Autodesk Fusion 360 part; units mm, degrees
(part 4 of 5)
sketch "Skizze60" plane through (0, 0, 0) normal (0, -1, 0) x (1, 0, 0)
  arc A0 (-6.1259, 60.1453) -> (-6.4721, 59.7023) centre (0, 55) ccw
  arc A1 (-6.4721, 59.7023) -> (-6.8553, 59.1236) centre (-6.6397, 59.397) ccw
  arc A2 (-6.8553, 59.1236) -> (-7.1281, 58.6319) centre (0, 55) ccw
  arc A3 (-7.1281, 58.6319) -> (-7.416, 58.0005) centre (-7.2458, 58.3042) ccw
  arc A4 (-7.416, 58.0005) -> (-7.6085, 57.4721) centre (0, 55) ccw
  arc A5 (-7.6085, 57.4721) -> (-7.7941, 56.8034) centre (-7.6734, 57.13) ccw
  arc A6 (-7.7941, 56.8034) -> (-7.9015, 56.2515) centre (0, 55) ccw
  arc A7 (-7.9015, 56.2515) -> (-7.9802, 55.5619) centre (-7.9122, 55.9034) ccw
  arc A8 (-7.9802, 55.5619) -> (-8, 55) centre (0, 55) ccw
  arc A9 (-8, 55) -> (-7.9699, 54.3066) centre (-7.9561, 54.6546) ccw
  arc A10 (-7.9699, 54.3066) -> (-7.9015, 53.7485) centre (0, 55) ccw
  arc A11 (-7.9015, 53.7485) -> (-7.7633, 53.0684) centre (-7.8041, 53.4142) ccw
  arc A12 (-7.7633, 53.0684) -> (-7.6085, 52.5279) centre (0, 55) ccw
  arc A13 (-7.6085, 52.5279) -> (-7.3656, 51.8777) centre (-7.46, 52.2129) ccw
  arc A14 (-7.3656, 51.8777) -> (-7.1281, 51.3681) centre (0, 55) ccw
  arc A15 (-7.1281, 51.3681) -> (-6.7864, 50.764) centre (-6.9321, 51.0802) ccw
  arc A16 (-6.7864, 50.764) -> (-6.4721, 50.2977) centre (0, 55) ccw
  arc A17 (-6.4721, 50.2977) -> (-6.0402, 49.7545) centre (-6.2336, 50.0441) ccw
  arc A18 (-6.0402, 49.7545) -> (-5.6569, 49.3431) centre (0, 55) ccw
  arc A19 (-5.6569, 49.3431) -> (-5.1453, 48.8741) centre (-5.3816, 49.1299) ccw
  arc A20 (-5.1453, 48.8741) -> (-4.7023, 48.5279) centre (0, 55) ccw
  arc A21 (-4.7023, 48.5279) -> (-4.1236, 48.1447) centre (-4.397, 48.3603) ccw
  arc A22 (-4.1236, 48.1447) -> (-3.6319, 47.8719) centre (0, 55) ccw
  arc A23 (-3.6319, 47.8719) -> (-3.0005, 47.584) centre (-3.3042, 47.7542) ccw
  arc A24 (-3.0005, 47.584) -> (-2.4721, 47.3915) centre (0, 55) ccw
  arc A25 (-2.4721, 47.3915) -> (-1.8034, 47.2059) centre (-2.13, 47.3266) ccw
  arc A26 (-1.8034, 47.2059) -> (-1.2515, 47.0985) centre (0, 55) ccw
  arc A27 (-1.2515, 47.0985) -> (-0.5619, 47.0198) centre (-0.9034, 47.0878) ccw
  arc A28 (-0.5619, 47.0198) -> (0, 47) centre (0, 55) ccw
  arc A29 (0, 47) -> (0.6934, 47.0301) centre (0.3454, 47.0439) ccw
  arc A30 (0.6934, 47.0301) -> (1.2515, 47.0985) centre (0, 55) ccw
  arc A31 (1.2515, 47.0985) -> (1.9316, 47.2367) centre (1.5858, 47.1959) ccw
  arc A32 (1.9316, 47.2367) -> (2.4721, 47.3915) centre (0, 55) ccw
  arc A33 (2.4721, 47.3915) -> (3.1223, 47.6344) centre (2.7871, 47.54) ccw
  arc A34 (3.1223, 47.6344) -> (3.6319, 47.8719) centre (0, 55) ccw
  arc A35 (3.6319, 47.8719) -> (4.236, 48.2136) centre (3.9198, 48.0679) ccw
  arc A36 (4.236, 48.2136) -> (4.7023, 48.5279) centre (0, 55) ccw
  arc A37 (4.7023, 48.5279) -> (5.2455, 48.9598) centre (4.9559, 48.7664) ccw
  arc A38 (5.2455, 48.9598) -> (5.6569, 49.3431) centre (0, 55) ccw
  arc A39 (5.6569, 49.3431) -> (6.1259, 49.8547) centre (5.8701, 49.6184) ccw
  arc A40 (6.1259, 49.8547) -> (6.4721, 50.2977) centre (0, 55) ccw
  arc A41 (6.4721, 50.2977) -> (6.8553, 50.8764) centre (6.6397, 50.603) ccw
  arc A42 (6.8553, 50.8764) -> (7.1281, 51.3681) centre (0, 55) ccw
  arc A43 (7.1281, 51.3681) -> (7.416, 51.9995) centre (7.2458, 51.6958) ccw
  arc A44 (7.416, 51.9995) -> (7.6085, 52.5279) centre (0, 55) ccw
  arc A45 (7.6085, 52.5279) -> (7.7941, 53.1966) centre (7.6734, 52.87) ccw
  arc A46 (7.7941, 53.1966) -> (7.9015, 53.7485) centre (0, 55) ccw
  arc A47 (7.9015, 53.7485) -> (7.9802, 54.4381) centre (7.9122, 54.0966) ccw
  arc A48 (7.9802, 54.4381) -> (8, 55) centre (0, 55) ccw
  arc A49 (8, 55) -> (7.9699, 55.6934) centre (7.9561, 55.3454) ccw
  arc A50 (7.9699, 55.6934) -> (7.9015, 56.2515) centre (0, 55) ccw
  arc A51 (7.9015, 56.2515) -> (7.7633, 56.9316) centre (7.8041, 56.5858) ccw
  arc A52 (7.7633, 56.9316) -> (7.6085, 57.4721) centre (0, 55) ccw
  arc A53 (7.6085, 57.4721) -> (7.3656, 58.1223) centre (7.46, 57.7871) ccw
  arc A54 (7.3656, 58.1223) -> (7.1281, 58.6319) centre (0, 55) ccw
  arc A55 (7.1281, 58.6319) -> (6.7864, 59.236) centre (6.9321, 58.9198) ccw
  arc A56 (6.7864, 59.236) -> (6.4721, 59.7023) centre (0, 55) ccw
  arc A57 (6.4721, 59.7023) -> (6.0402, 60.2455) centre (6.2336, 59.9559) ccw
  arc A58 (6.0402, 60.2455) -> (5.6569, 60.6569) centre (0, 55) ccw
  arc A59 (5.6569, 60.6569) -> (5.1453, 61.1259) centre (5.3816, 60.8701) ccw
  arc A60 (5.1453, 61.1259) -> (4.7023, 61.4721) centre (0, 55) ccw
  arc A61 (4.7023, 61.4721) -> (4.1236, 61.8553) centre (4.397, 61.6397) ccw
  arc A62 (4.1236, 61.8553) -> (3.6319, 62.1281) centre (0, 55) ccw
  arc A63 (3.6319, 62.1281) -> (3.0005, 62.416) centre (3.3042, 62.2458) ccw
  arc A64 (3.0005, 62.416) -> (2.4721, 62.6085) centre (0, 55) ccw
  arc A65 (2.4721, 62.6085) -> (1.8034, 62.7941) centre (2.13, 62.6734) ccw
  arc A66 (1.8034, 62.7941) -> (1.2515, 62.9015) centre (0, 55) ccw
  arc A67 (1.2515, 62.9015) -> (0.5619, 62.9802) centre (0.9034, 62.9122) ccw
  arc A68 (0.5619, 62.9802) -> (0, 63) centre (0, 55) ccw
  arc A69 (0, 63) -> (-0.6934, 62.9699) centre (-0.3454, 62.9561) ccw
  arc A70 (-0.6934, 62.9699) -> (-1.2515, 62.9015) centre (0, 55) ccw
  arc A71 (-1.2515, 62.9015) -> (-1.9316, 62.7633) centre (-1.5858, 62.8041) ccw
  arc A72 (-1.9316, 62.7633) -> (-2.4721, 62.6085) centre (0, 55) ccw
  arc A73 (-2.4721, 62.6085) -> (-3.1223, 62.3656) centre (-2.7871, 62.46) ccw
  arc A74 (-3.1223, 62.3656) -> (-3.6319, 62.1281) centre (0, 55) ccw
  arc A75 (-3.6319, 62.1281) -> (-4.236, 61.7864) centre (-3.9198, 61.9321) ccw
  arc A76 (-4.236, 61.7864) -> (-4.7023, 61.4721) centre (0, 55) ccw
  arc A77 (-4.7023, 61.4721) -> (-5.2455, 61.0402) centre (-4.9559, 61.2336) ccw
  arc A78 (-5.2455, 61.0402) -> (-5.6569, 60.6569) centre (0, 55) ccw
  arc A79 (-5.6569, 60.6569) -> (-6.1259, 60.1453) centre (-5.8701, 60.3816) ccw
  circle A80 centre (0, 55) radius 8
  constraint concentric A0 A80
extrude "Extrusion65" add sketch "Skizze60" along normal blind 1 contours A0 A2 A4 A6 A8 A10 A12 A14 A16 A18 A20 A22 A24 A26 A28 A30 A32 A34 A36 A38 A40 A42 A44 A46 A48 A50 A52 A54 A56 A58 A60 A62 A64 A66 A68 A70 A72 A74 A76 A78 A80 bodies 3
chamfer "Fase2" distance 1 angle 45 1 edges at (-7.4586, -1, 52.1071) on bodies 3
sketch "Skizze61" plane through (0, 0, 27.5) normal (0, 0, 1) x (1, 0, 0)
  line L0 (-32.5, 0) -> (32.5, 0)
  line L1 (32.5, 0) -> (32.5, 16)
  line L2 (32.5, 16) -> (-32.5, 16)
  line L3 (-32.5, 16) -> (-32.5, 0)
  line L4 (-9.4118, 6.9027) -> (-15.8397, 14.5631)
  arc A0 (-15.8397, 14.5631) -> (-18.1378, 12.6348) centre (-16.9888, 13.599) ccw
  line L5 (-18.1378, 12.6348) -> (-11.71, 4.9743)
  arc A1 (-11.71, 4.9743) -> (-9.4118, 6.9027) centre (-10.5609, 5.9385) ccw
  line L6 (-10.5609, 5.9385) -> (-16.9888, 13.599) construction
  line L7 (-9.1378, 12.6348) -> (-2.71, 4.9743)
  arc A2 (-6.8397, 14.5631) -> (-9.1378, 12.6348) centre (-7.9888, 13.599) ccw
  line L8 (-0.4118, 6.9027) -> (-6.8397, 14.5631)
  arc A3 (-2.71, 4.9743) -> (-0.4118, 6.9027) centre (-1.5609, 5.9385) ccw
  line L9 (-0.1378, 12.6348) -> (6.29, 4.9743)
  arc A4 (2.1603, 14.5631) -> (-0.1378, 12.6348) centre (1.0112, 13.599) ccw
  line L10 (8.5882, 6.9027) -> (2.1603, 14.5631)
  arc A5 (6.29, 4.9743) -> (8.5882, 6.9027) centre (7.4391, 5.9385) ccw
  line L11 (8.8622, 12.6348) -> (15.29, 4.9743)
  arc A6 (11.1603, 14.5631) -> (8.8622, 12.6348) centre (10.0112, 13.599) ccw
  line L12 (17.5882, 6.9027) -> (11.1603, 14.5631)
  arc A7 (15.29, 4.9743) -> (17.5882, 6.9027) centre (16.4391, 5.9385) ccw
  dimension "d317" = 3
  dimension "d320" = 27
  dimension "d321" = 0
  constraint tangent L4 A0
  constraint tangent A0 L5
  constraint parallel L4 L5
  constraint tangent L5 A1
  constraint tangent L4 A1
  measures "d317" diameter of A0
extrude "Extrusion66" cut sketch "Skizze61" against normal blind 2 contours L4 A0 L5 A1 | L7 A2 L8 A3 | L9 A4 L10 A5 | L11 A6 L12 A7 bodies 1
extrude "Extrusion67" cut 1 faces at (0.4189, 1, 54.1158) along direction (0, -1, 0) blind 1 on bodies 3 bodies 3
sketch "Skizze62" plane through (0, 10.5, 0) normal (0, 1, 0) x (-1, 0, 0)
  arc A0 (-3.1, 55) -> (1.4484, 57.7408) centre (0, 55) ccw
  line L0 (-3.1, 55) -> (1.4484, 57.7408)
  circle A1 centre (0, 55) radius 4.5
  circle A2 centre (0, 55) radius 3.1
  constraint concentric A0 A2
extrude "Extrusion68" add sketch "Skizze62" along normal blind 3 bodies 3
sketch "Skizze63" plane through (0, 47, 0) normal (0, 1, 0) x (-1, 0, 0)
  line L0 (-20.5, -7.58) -> (-20.5, -6.3514)
  arc A0 (-20.5, -4.3514) -> (-20.5, -6.3514) centre (-20.5, -5.3514) ccw
  line L1 (-20.5, -4.3514) -> (-12.5, -4.3514)
  arc A1 (-12.5, -6.3514) -> (-12.5, -4.3514) centre (-12.5, -5.3514) ccw
  line L2 (-12.5, -6.3514) -> (-12.5, -7.58)
  line L3 (-12.5, -7.58) -> (-20.5, -7.58)
  circle A2 centre (3.5, 16) radius 6.5
  line L4 (21.5, -1.5) -> (21.5, -23.5)
  line L5 (21.5, -23.5) -> (-5.5, -23.5)
  line L6 (-5.5, -23.5) -> (-5.5, -1.5)
  line L7 (-5.5, -1.5) -> (21.5, -1.5)
  line L8 (-37.3325, 4.5) -> (-48.5, 4.5)
  arc A3 (-48.5, 7.5) -> (-48.5, 4.5) centre (-48.5, 6) ccw
  line L9 (-48.5, 7.5) -> (-37.3325, 7.5)
  arc A4 (-37.3325, 4.5) -> (-37.3325, 7.5) centre (-37.3325, 6) ccw
  line L10 (-12.5, 2.5057) -> (-20.5, 2.5057)
  arc A5 (-20.5, 4.5057) -> (-20.5, 2.5057) centre (-20.5, 3.5057) ccw
  line L11 (-20.5, 4.5057) -> (-12.5, 4.5057)
  arc A6 (-12.5, 2.5057) -> (-12.5, 4.5057) centre (-12.5, 3.5057) ccw
  line L12 (-12.5, -15.2086) -> (-20.5, -15.2086)
  arc A7 (-20.5, -13.2086) -> (-20.5, -15.2086) centre (-20.5, -14.2086) ccw
  line L13 (-20.5, -13.2086) -> (-12.5, -13.2086)
  arc A8 (-12.5, -15.2086) -> (-12.5, -13.2086) centre (-12.5, -14.2086) ccw
  arc A9 (34, 7.5) -> (34, 4.5) centre (34, 6) ccw
  line L14 (34, 7.5) -> (45, 7.5)
  arc A10 (45, 4.5) -> (45, 7.5) centre (45, 6) ccw
  line L15 (45, 4.5) -> (34, 4.5)
  arc A11 (34, -10.5) -> (34, -13.5) centre (34, -12) ccw
  line L16 (34, -10.5) -> (45, -10.5)
  arc A12 (45, -13.5) -> (45, -10.5) centre (45, -12) ccw
  line L17 (45, -13.5) -> (34, -13.5)
  arc A13 (34, 13.5) -> (34, 10.5) centre (34, 12) ccw
  line L18 (34, 13.5) -> (45, 13.5)
  arc A14 (45, 10.5) -> (45, 13.5) centre (45, 12) ccw
  line L19 (45, 10.5) -> (34, 10.5)
  line L20 (-12.5, -10.78) -> (-20.5, -10.78)
  arc A15 (-20.5, -8.78) -> (-20.5, -10.78) centre (-20.5, -9.78) ccw
  line L21 (-20.5, -8.78) -> (-12.5, -8.78)
  arc A16 (-12.5, -10.78) -> (-12.5, -8.78) centre (-12.5, -9.78) ccw
  line L22 (-20.5, 8.9343) -> (-12.5, 8.9343)
  arc A17 (-12.5, 6.9343) -> (-12.5, 8.9343) centre (-12.5, 7.9343) ccw
  line L23 (-12.5, 6.9343) -> (-20.5, 6.9343)
  arc A18 (-20.5, 8.9343) -> (-20.5, 6.9343) centre (-20.5, 7.9343) ccw
  line L24 (-37.3325, -1.5) -> (-48.5, -1.5)
  arc A19 (-48.5, 1.5) -> (-48.5, -1.5) centre (-48.5, 0) ccw
  line L25 (-48.5, 1.5) -> (-37.3325, 1.5)
  arc A20 (-37.3325, -1.5) -> (-37.3325, 1.5) centre (-37.3325, 0) ccw
  arc A21 (-20.8852, 0) -> (-20.5, -1.9228) centre (-20.5, -0.9228) ccw
  line L26 (-20.8852, 0) -> (-12.1148, 0)
  arc A22 (-12.5, -1.9228) -> (-12.1148, 0) centre (-12.5, -0.9228) ccw
  line L27 (-12.5, -1.9228) -> (-20.5, -1.9228)
  line L28 (-12.5, -19.6371) -> (-20.5, -19.6371)
  arc A23 (-20.5, -17.6371) -> (-20.5, -19.6371) centre (-20.5, -18.6371) ccw
  line L29 (-20.5, -17.6371) -> (-12.5, -17.6371)
  arc A24 (-12.5, -19.6371) -> (-12.5, -17.6371) centre (-12.5, -18.6371) ccw
  line L30 (34, 1.5) -> (45, 1.5)
  arc A25 (45, -1.5) -> (45, 1.5) centre (45, 0) ccw
  line L31 (45, -1.5) -> (34, -1.5)
  arc A26 (34, 1.5) -> (34, -1.5) centre (34, 0) ccw
  arc A27 (34, -4.5) -> (34, -7.5) centre (34, -6) ccw
  line L32 (34, -4.5) -> (45, -4.5)
  arc A28 (45, -7.5) -> (45, -4.5) centre (45, -6) ccw
  line L33 (45, -7.5) -> (34, -7.5)
  line L34 (-12.5, -24.0657) -> (-20.5, -24.0657)
  arc A29 (-20.5, -22.0657) -> (-20.5, -24.0657) centre (-20.5, -23.0657) ccw
  line L35 (-20.5, -22.0657) -> (-12.5, -22.0657)
  arc A30 (-12.5, -24.0657) -> (-12.5, -22.0657) centre (-12.5, -23.0657) ccw
  line L36 (-37.3325, -7.5) -> (-48.5, -7.5)
  arc A31 (-48.5, -4.5) -> (-48.5, -7.5) centre (-48.5, -6) ccw
  line L37 (-48.5, -4.5) -> (-37.3325, -4.5)
  arc A32 (-37.3325, -7.5) -> (-37.3325, -4.5) centre (-37.3325, -6) ccw
  line L38 (22.3, -10.5) -> (30, -10.5)
  line L39 (30, -10.5) -> (30, -18.5)
  line L40 (30, -18.5) -> (22.3, -18.5)
  line L41 (22.3, -18.5) -> (22.3, -10.5)
  line L42 (-32.5, 27.5) -> (-32.5, 14.5)
  arc A33 (-36, 11) -> (-32.5, 14.5) centre (-36, 14.5) ccw
  line L43 (-36, 11) -> (-56.5, 11)
  line L44 (-56.5, 11) -> (-56.5, -11)
  line L45 (-56.5, -11) -> (-36, -11)
  arc A34 (-32.5, -14.5) -> (-36, -11) centre (-36, -14.5) ccw
  line L46 (-32.5, -14.5) -> (-32.5, -27.5)
  line L47 (-32.5, -27.5) -> (32, -27.5)
  line L48 (32, -27.5) -> (32, -25)
  arc A35 (36, -21) -> (32, -25) centre (36, -25) ccw
  line L49 (36, -21) -> (43, -21)
  line L50 (43, -21) -> (57.5, -6.5)
  line L51 (57.5, -6.5) -> (57.5, 6.5)
  line L52 (57.5, 6.5) -> (43, 21)
  line L53 (43, 21) -> (36, 21)
  arc A36 (32, 25) -> (36, 21) centre (36, 25) ccw
  line L54 (32, 25) -> (32, 27.5)
  line L55 (32, 27.5) -> (-10.5, 27.5)
  line L56 (-10.5, 27.5) -> (-10.5, 21.5)
  line L57 (-10.5, 21.5) -> (-12, 21.5)
  line L58 (-12, 21.5) -> (-12, 11.5)
  line L59 (-12, 11.5) -> (-21, 11.5)
  line L60 (-21, 11.5) -> (-21, 21.5)
  line L61 (-21, 21.5) -> (-22.5, 21.5)
  line L62 (-22.5, 21.5) -> (-22.5, 27.5)
  line L63 (-20.5, -22.0657) -> (-12.5, -22.0657)
  line L64 (-12.5, -19.6371) -> (-20.5, -19.6371)
  line L65 (-12.5, -22.0657) -> (-12.5, -19.6371)
  line L66 (-20.5, -22.0657) -> (-20.5, -19.6371)
  line L67 (-22.5, 27.5) -> (-32.5, 27.5)
  constraint coincident L35.end A30.end
  constraint coincident L28.start A24.start
  constraint coincident A29.start L35.start
  constraint coincident L28.end A23.end
extrude "Extrusion69" cut sketch "Skizze63" against normal blind 1 contours L28 L35 L63 L64 L65 L66 bodies 2
sketch "Skizze64" plane through (0, 0, -27.5) normal (0, 0, -1) x (-1, 0, 0)
  arc A0 (12.7093, 36.1235) -> (-12.7093, 36.1235) centre (0, 22) ccw
  line L0 (12.7093, 36.1235) -> (0.5176, 23.9319)
  arc A1 (0.5176, 23.9319) -> (-0.5176, 23.9319) centre (0, 22) ccw
  line L1 (-0.5176, 23.9319) -> (-12.7093, 36.1235)
  circle A2 centre (16, 38) radius 1.75
  circle A3 centre (-16, 38) radius 1.75
  line L2 (-13, 44) -> (-13, 42)
  line L3 (-13, 42) -> (-20, 42)
  line L4 (-20, 42) -> (-20, 35.2606)
  line L5 (-20, 35.2606) -> (-22, 35.2606)
  line L6 (-22, 35.2606) -> (-22, 44)
  line L7 (13, 44) -> (22, 44)
  line L8 (-32.5, 47) -> (-32.5, 16)
  line L9 (18.0278, 16) -> (32.5, 16)
  arc A4 (-14.1235, 34.7093) -> (-18.0278, 16) centre (0, 22) ccw
  line L10 (-14.1235, 34.7093) -> (-1.9319, 22.5176)
  arc A5 (-1.9319, 22.5176) -> (-1.9319, 21.4824) centre (0, 22) ccw
  line L11 (-1.9319, 21.4824) -> (-7.4142, 16)
  line L12 (-7.4142, 16) -> (-4.5858, 16)
  line L13 (-4.5858, 16) -> (-0.5176, 20.0681)
  arc A6 (-0.5176, 20.0681) -> (0.5176, 20.0681) centre (0, 22) ccw
  line L14 (0.5176, 20.0681) -> (4.5858, 16)
  line L15 (4.5858, 16) -> (7.4142, 16)
  line L16 (7.4142, 16) -> (1.9319, 21.4824)
  arc A7 (1.9319, 21.4824) -> (1.9319, 22.5176) centre (0, 22) ccw
  line L17 (1.9319, 22.5176) -> (14.1235, 34.7093)
  arc A8 (18.0278, 16) -> (14.1235, 34.7093) centre (0, 22) ccw
  line L18 (32.5, 19) -> (32.5, 33.5)
  line L19 (32.5, 33.5) -> (32, 33.5)
  line L20 (32, 33.5) -> (32, 47)
  line L21 (22, 44) -> (22, 35)
  line L22 (22, 35) -> (20.1, 35)
  line L23 (20.1, 35) -> (20.1, 42)
  line L24 (20.1, 42) -> (13, 42)
  line L25 (13, 42) -> (13, 44)
  line L26 (4.5858, 16) -> (0.5176, 20.0681)
  arc A9 (-0.5176, 20.0681) -> (0.5176, 20.0681) centre (0, 22) ccw
  line L27 (-0.5176, 20.0681) -> (-4.5858, 16)
  line L28 (-4.5858, 16) -> (-7.4142, 16)
  line L29 (-7.4142, 16) -> (-1.9319, 21.4824)
  arc A10 (-1.9319, 22.5176) -> (-1.9319, 21.4824) centre (0, 22) ccw
  line L30 (-1.9319, 22.5176) -> (-14.1235, 34.7093)
  arc A11 (-14.1235, 34.7093) -> (-18.0278, 16) centre (0, 22) ccw
  line L31 (-18.0278, 16) -> (-23, 16)
  line L32 (-23, 16) -> (-23, 45)
  line L33 (-23, 45) -> (23, 45)
  line L34 (23, 45) -> (23, 16)
  line L35 (23, 16) -> (18.0278, 16)
  arc A12 (18.0278, 16) -> (14.1235, 34.7093) centre (0, 22) ccw
  line L36 (14.1235, 34.7093) -> (1.9319, 22.5176)
  arc A13 (1.9319, 21.4824) -> (1.9319, 22.5176) centre (0, 22) ccw
  line L37 (1.9319, 21.4824) -> (7.4142, 16)
  line L38 (7.4142, 16) -> (4.5858, 16)
  arc A14 (12.7093, 36.1235) -> (-12.7093, 36.1235) centre (0, 22) ccw
  line L39 (-12.7093, 36.1235) -> (-0.5176, 23.9319)
  arc A15 (0.5176, 23.9319) -> (-0.5176, 23.9319) centre (0, 22) ccw
  line L40 (0.5176, 23.9319) -> (12.7093, 36.1235)
  circle A16 centre (16, 38) radius 1.75
  circle A17 centre (-16, 38) radius 1.75
  circle A18 centre (0, 22) radius 19
  line L41 (-22, 44) -> (-13, 44)
  line L42 (32.5, 16) -> (32.5, 19)
  line L43 (32, 47) -> (-32.5, 47)
  line L44 (-32.5, 16) -> (-18.0278, 16)
  constraint concentric A9 A18
extrude "Extrusion70" cut sketch "Skizze64" against normal blind 2 contours L0 A1 L1 L10 A5 L11 L12 L13 A6 L14 L15 L16 A7 L17 L26 A9 L27 L28 L29 A10 L30 L36 A13 L37 L38 L39 A15 L40 A18 | A4 L10 A5 L11 L12 L13 A6 L14 L15 L16 A7 L17 A8 L26 A9 L27 L28 L29 A10 L30 A11 A12 L36 A13 L37 L38 A18 bodies 1 2
sketch "Skizze65" plane through (0, 0, -27.5) normal (0, 0, -1) x (-1, 0, 0)
  arc A0 (18.0278, 16) -> (-18.0278, 16) centre (0, 22) ccw
  line L0 (18.0278, 16) -> (32.5, 16)
  line L1 (32.5, 19) -> (32.5, 33.5)
  line L2 (32.5, 33.5) -> (32, 33.5)
  line L3 (32, 33.5) -> (32, 47)
  line L4 (32, 47) -> (-32.5, 47)
  line L5 (22, 44) -> (22, 35)
  line L6 (22, 35) -> (20.1, 35)
  line L7 (20.1, 35) -> (20.1, 42)
  line L8 (20.1, 42) -> (13, 42)
  line L9 (13, 42) -> (13, 44)
  line L10 (-13, 44) -> (-13, 42)
  line L11 (-13, 42) -> (-20, 42)
  line L12 (-20, 42) -> (-20, 35.2606)
  line L13 (-20, 35.2606) -> (-22, 35.2606)
  line L14 (-22, 35.2606) -> (-22, 44)
  line L15 (-32.5, 47) -> (-32.5, 16)
  line L16 (-32.5, 16) -> (-18.0278, 16)
  circle A1 centre (16, 38) radius 1.75
  circle A2 centre (-16, 38) radius 1.75
  circle A3 centre (-16, 38) radius 1.75
  circle A4 centre (16, 38) radius 1.75
  circle A5 centre (-16, 6) radius 1.75
  line L17 (32.5, 16) -> (32.5, 19)
  line L18 (13, 44) -> (22, 44)
  line L19 (-22, 44) -> (-13, 44)
  point P0 (14.25, 38)
extrude "Extrusion71" add sketch "Skizze65" against normal blind 1.5 contours A1 A4 | A2 A3 | A5 bodies 1 2
chamfer "Fase3" distance 0.5 angle 45 1 edges at (2.8902, 13.5, 56.121) on bodies 3
sketch "Skizze66" plane through (0, 21.5, 0) normal (0, -1, 0) x (1, 0, 0)
  line L0 (56.5, -5) -> (51.5, -5)
  line L1 (51.5, -5) -> (51.5, -9.5)
  line L2 (51.5, -9.5) -> (31, -9.5)
  line L3 (31, -9.5) -> (31, -19.2)
  line L4 (31, -19.2) -> (32.5, -19.2)
  line L5 (32.5, -19.2) -> (32.5, -19)
  arc A0 (33.5, -18) -> (32.5, -19) centre (33.5, -19) ccw
  line L6 (33.5, -18) -> (38.5, -18)
  arc A1 (38.5, -18) -> (39.5, -17) centre (38.5, -17) ccw
  line L7 (39.5, -17) -> (39.5, -12)
  arc A2 (40.5, -11) -> (39.5, -12) centre (40.5, -12) ccw
  line L8 (40.5, -11) -> (56.5, -11)
  line L9 (56.5, -11) -> (56.5, -5)
  circle A3 centre (36, -14.5) radius 1.9
  line L10 (56.5, 5) -> (56.5, -5)
  line L11 (56.5, 5) -> (51.5, 5)
  line L12 (51.5, -5) -> (51.5, 5)
  line L13 (51.5, -5) -> (56.5, -5)
  circle A4 centre (-3.5, 16) radius 6.5
  line L14 (-21.5, -1.5) -> (-21.5, -23.5)
  line L15 (-21.5, -23.5) -> (5.5, -23.5)
  line L16 (5.5, -23.5) -> (5.5, -1.5)
  line L17 (5.5, -1.5) -> (-21.5, -1.5)
  line L18 (37.3325, 4.5) -> (48.5, 4.5)
  arc A5 (48.5, 4.5) -> (48.5, 7.5) centre (48.5, 6) ccw
  line L19 (48.5, 7.5) -> (37.3325, 7.5)
  arc A6 (37.3325, 7.5) -> (37.3325, 4.5) centre (37.3325, 6) ccw
  line L20 (12.5, 2.5057) -> (20.5, 2.5057)
  arc A7 (20.5, 2.5057) -> (20.5, 4.5057) centre (20.5, 3.5057) ccw
  line L21 (20.5, 4.5057) -> (12.5, 4.5057)
  arc A8 (12.5, 4.5057) -> (12.5, 2.5057) centre (12.5, 3.5057) ccw
  line L22 (12.5, -15.2086) -> (20.5, -15.2086)
  arc A9 (20.5, -15.2086) -> (20.5, -13.2086) centre (20.5, -14.2086) ccw
  line L23 (20.5, -13.2086) -> (12.5, -13.2086)
  arc A10 (12.5, -13.2086) -> (12.5, -15.2086) centre (12.5, -14.2086) ccw
  arc A11 (-34, 4.5) -> (-34, 7.5) centre (-34, 6) ccw
  line L24 (-34, 7.5) -> (-45, 7.5)
  arc A12 (-45, 7.5) -> (-45, 4.5) centre (-45, 6) ccw
  line L25 (-45, 4.5) -> (-34, 4.5)
  arc A13 (-34, -13.5) -> (-34, -10.5) centre (-34, -12) ccw
  line L26 (-34, -10.5) -> (-45, -10.5)
  arc A14 (-45, -10.5) -> (-45, -13.5) centre (-45, -12) ccw
  line L27 (-45, -13.5) -> (-34, -13.5)
  arc A15 (-34, 10.5) -> (-34, 13.5) centre (-34, 12) ccw
  line L28 (-34, 13.5) -> (-45, 13.5)
  arc A16 (-45, 13.5) -> (-45, 10.5) centre (-45, 12) ccw
  line L29 (-45, 10.5) -> (-34, 10.5)
  line L30 (12.5, -10.78) -> (20.5, -10.78)
  arc A17 (20.5, -10.78) -> (20.5, -8.78) centre (20.5, -9.78) ccw
  line L31 (20.5, -8.78) -> (12.5, -8.78)
  arc A18 (12.5, -8.78) -> (12.5, -10.78) centre (12.5, -9.78) ccw
  line L32 (20.5, 8.9343) -> (12.5, 8.9343)
  arc A19 (12.5, 8.9343) -> (12.5, 6.9343) centre (12.5, 7.9343) ccw
  line L33 (12.5, 6.9343) -> (20.5, 6.9343)
  arc A20 (20.5, 6.9343) -> (20.5, 8.9343) centre (20.5, 7.9343) ccw
  line L34 (37.3325, -1.5) -> (48.5, -1.5)
  arc A21 (48.5, -1.5) -> (48.5, 1.5) centre (48.5, 0) ccw
  line L35 (48.5, 1.5) -> (37.3325, 1.5)
  arc A22 (37.3325, 1.5) -> (37.3325, -1.5) centre (37.3325, 0) ccw
  arc A23 (20.5, -1.9228) -> (20.8852, 0) centre (20.5, -0.9228) ccw
  line L36 (20.8852, 0) -> (12.1148, 0)
  arc A24 (12.1148, 0) -> (12.5, -1.9228) centre (12.5, -0.9228) ccw
  line L37 (12.5, -1.9228) -> (20.5, -1.9228)
  line L38 (20.5, -22.0657) -> (20.5, -19.6371)
  arc A25 (20.5, -19.6371) -> (20.5, -17.6371) centre (20.5, -18.6371) ccw
  line L39 (20.5, -17.6371) -> (12.5, -17.6371)
  arc A26 (12.5, -17.6371) -> (12.5, -19.6371) centre (12.5, -18.6371) ccw
  line L40 (12.5, -19.6371) -> (12.5, -22.0657)
  arc A27 (12.5, -22.0657) -> (12.5, -24.0657) centre (12.5, -23.0657) ccw
  line L41 (12.5, -24.0657) -> (20.5, -24.0657)
  arc A28 (20.5, -24.0657) -> (20.5, -22.0657) centre (20.5, -23.0657) ccw
  line L42 (-34, 1.5) -> (-45, 1.5)
  arc A29 (-45, 1.5) -> (-45, -1.5) centre (-45, 0) ccw
  line L43 (-45, -1.5) -> (-34, -1.5)
  arc A30 (-34, -1.5) -> (-34, 1.5) centre (-34, 0) ccw
  arc A31 (-34, -7.5) -> (-34, -4.5) centre (-34, -6) ccw
  line L44 (-34, -4.5) -> (-45, -4.5)
  arc A32 (-45, -4.5) -> (-45, -7.5) centre (-45, -6) ccw
  line L45 (-45, -7.5) -> (-34, -7.5)
  line L46 (37.3325, -7.5) -> (48.5, -7.5)
  arc A33 (48.5, -7.5) -> (48.5, -4.5) centre (48.5, -6) ccw
  line L47 (48.5, -4.5) -> (37.3325, -4.5)
  arc A34 (37.3325, -4.5) -> (37.3325, -7.5) centre (37.3325, -6) ccw
  line L48 (-22.3, -10.5) -> (-30, -10.5)
  line L49 (-30, -10.5) -> (-30, -18.5)
  line L50 (-30, -18.5) -> (-22.3, -18.5)
  line L51 (-22.3, -18.5) -> (-22.3, -10.5)
  line L52 (36, 11) -> (56.5, 11)
  line L53 (56.5, 11) -> (56.5, -11)
  line L54 (56.5, -11) -> (36, -11)
  arc A35 (36, -11) -> (32.5, -14.5) centre (36, -14.5) ccw
  line L55 (32.5, -14.5) -> (32.5, -27.5)
  line L56 (32.5, -27.5) -> (-32, -27.5)
  line L57 (-32, -27.5) -> (-32, -25)
  arc A36 (-32, -25) -> (-36, -21) centre (-36, -25) ccw
  line L58 (-36, -21) -> (-43, -21)
  line L59 (-43, -21) -> (-57.5, -6.5)
  line L60 (-57.5, -6.5) -> (-57.5, 6.5)
  line L61 (-57.5, 6.5) -> (-43, 21)
  line L62 (-43, 21) -> (-36, 21)
  arc A37 (-36, 21) -> (-32, 25) centre (-36, 25) ccw
  line L63 (-32, 25) -> (-32, 27.5)
  line L64 (-32, 27.5) -> (10.5, 27.5)
  line L65 (10.5, 27.5) -> (10.5, 21.5)
  line L66 (10.5, 21.5) -> (12, 21.5)
  line L67 (12, 21.5) -> (12, 11.5)
  line L68 (12, 11.5) -> (21, 11.5)
  line L69 (21, 11.5) -> (21, 21.5)
  line L70 (21, 21.5) -> (22.5, 21.5)
  line L71 (22.5, 21.5) -> (22.5, 27.5)
  line L72 (22.5, 27.5) -> (32.5, 27.5)
  line L73 (32.5, 27.5) -> (32.5, 14.5)
  arc A38 (32.5, 14.5) -> (36, 11) centre (36, 14.5) ccw
  line L74 (20.5, -7.58) -> (20.5, -6.3514)
  arc A39 (20.5, -6.3514) -> (20.5, -4.3514) centre (20.5, -5.3514) ccw
  line L75 (20.5, -4.3514) -> (12.5, -4.3514)
  arc A40 (12.5, -4.3514) -> (12.5, -6.3514) centre (12.5, -5.3514) ccw
  line L76 (12.5, -6.3514) -> (12.5, -7.58)
  line L77 (12.5, -7.58) -> (20.5, -7.58)
  line L78 (51.5, 5) -> (56.5, 5)
  line L79 (56.5, 5) -> (56.5, 11)
  line L80 (56.5, 11) -> (40.5, 11)
  arc A41 (39.5, 12) -> (40.5, 11) centre (40.5, 12) ccw
  line L81 (39.5, 12) -> (39.5, 17)
  arc A42 (39.5, 17) -> (38.5, 18) centre (38.5, 17) ccw
  line L82 (38.5, 18) -> (33.5, 18)
  arc A43 (32.5, 19) -> (33.5, 18) centre (33.5, 19) ccw
  line L83 (32.5, 19) -> (32.5, 19.2)
  line L84 (32.5, 19.2) -> (31, 19.2)
  line L85 (31, 19.2) -> (31, 9.5)
  line L86 (31, 9.5) -> (51.5, 9.5)
  line L87 (51.5, 9.5) -> (51.5, 5)
  circle A44 centre (36, 14.5) radius 1.9
extrude "Extrusion72" cut sketch "Skizze66" against normal blind 3 contours L0 L1 L2 L3 L4 L5 L8 L9 L13 L53 L54 A35 L55 | L0 L10 L11 L12 L13 L53 L78 | L11 L52 L53 L73 A38 L78 L79 L80 L83 L84 L85 L86 L87 | A0 L6 A1 L7 A2 L54 A35 L55 | L52 L73 A38 A41 L81 A42 L82 A43 bodies 2
sketch "Skizze67" plane through (0, 16, 0) normal (0, -1, 0) x (1, 0, 0)
  circle A0 centre (-36, -25) radius 1.9
  line L0 (-18.0278, -27.5) -> (-18.0278, -26)
  line L1 (-18.0278, -26) -> (-23, -26)
  line L2 (-23, -26) -> (-31, -26)
  line L3 (-31, -26) -> (-31, -20)
  line L4 (-31, -20) -> (-41.8787, -20)
  line L5 (-41.8787, -20) -> (-51.5218, -10.3569)
  line L6 (-51.5218, -10.3569) -> (-51.5218, -5)
  line L7 (-51.5218, -5) -> (-57.5, -5)
  line L8 (-57.5, -5) -> (-57.5, -6.5)
  line L9 (-57.5, -6.5) -> (-42.5, -21.5)
  line L10 (-42.5, -21.5) -> (-38.922, -26.9266)
  arc A1 (-38.922, -26.9266) -> (-34.8649, -28.3108) centre (-36, -25) ccw
  line L11 (-34.8649, -28.3108) -> (-32.5, -27.5)
  line L12 (-32.5, -27.5) -> (-18.0278, -27.5)
  line L13 (-51.5218, 5) -> (-51.5218, -5)
  line L14 (-51.5218, 5) -> (-57.5, 5)
  line L15 (-57.5, -5) -> (-57.5, 5)
  line L16 (-57.5, -5) -> (-51.5218, -5)
  line L17 (-44.7071, 17.1716) -> (-47.5355, 14.3431)
  line L18 (-44.7071, 17.1716) -> (-45.7678, 18.2322)
  line L19 (-48.5962, 15.4038) -> (-45.7678, 18.2322)
  line L20 (-48.5962, 15.4038) -> (-47.5355, 14.3431)
extrude "Extrusion73" cut sketch "Skizze67" 3 faces at (-53.5145, 16, 7.2856) (-36.3402, 16, 21.0351) (24.5093, 16, -27) against normal blind 3 on bodies 2 bodies 2
extrude "Extrusion74" add 2 faces at (54.8333, 21.5, 8.5) (54.8333, 21.5, -8.5) along direction (0, 1, 0) blind 3 on bodies 1 bodies 1
extrude "Extrusion75" add 3 faces at (27.1759, 16, -27) (-53.5145, 16, 7.2856) (-53.5145, 16, -7.2856) along direction (0, 1, 0) blind 3 on bodies 1 bodies 1
sketch "Skizze68" plane through (0, 19, 0) normal (0, 1, 0) x (-1, 0, 0)
  line L0 (18.0278, -26) -> (18.0278, -27.5)
  line L1 (18.0278, -27.5) -> (32.5, -27.5)
  line L2 (32.5, -27.5) -> (33.8276, -28.3587)
  arc A0 (33.8276, -28.3587) -> (39.5022, -26.9326) centre (36, -25) ccw
  line L3 (39.5022, -26.9326) -> (42.5, -21.5)
  line L4 (42.5, -21.5) -> (57.5, -6.5)
  line L5 (57.5, -6.5) -> (57.5, -5)
  line L6 (57.5, -5) -> (51.5218, -5)
  line L7 (51.5218, -5) -> (51.5218, -10.3569)
  line L8 (51.5218, -10.3569) -> (41.8787, -20)
  line L9 (41.8787, -20) -> (31, -20)
  line L10 (31, -20) -> (31, -26)
  line L11 (31, -26) -> (18.0278, -26)
  circle A1 centre (36, -25) radius 1.9
  line L12 (51.5218, -5) -> (51.5218, 5)
  line L13 (51.5218, -5) -> (57.5, -5)
  line L14 (57.5, 5) -> (57.5, -5)
  line L15 (57.5, 5) -> (51.5218, 5)
  line L16 (-56.5, -5) -> (-56.5, 5)
  line L17 (-56.5, -5) -> (-51.5, -5)
  line L18 (-51.5, 5) -> (-51.5, -5)
  line L19 (-51.5, 5) -> (-56.5, 5)
  line L20 (-18.0278, -26) -> (0, -26)
  line L21 (-18.0278, -26) -> (-18.0278, -27.5)
  line L22 (18.0278, -27.5) -> (-18.0278, -27.5)
  line L23 (18.0278, -27.5) -> (18.0278, -26)
  line L24 (0, -26) -> (18.0278, -26)
extrude "Extrusion76" add sketch "Skizze68" against normal blind 17 contours L0 L20 L21 L22 L23 L24 | L6 L12 L13 L14 L15 bodies 1
sketch "Skizze69" plane through (0, 24.5, 0) normal (0, 1, 0) x (-1, 0, 0)
  circle A0 centre (-36, 14.5) radius 1.9
  arc A1 (-39.5, 18) -> (-40.5, 17) centre (-39.5, 17) ccw
  line L0 (-40.5, 17) -> (-40.5, 12)
  arc A2 (-41.5, 11) -> (-40.5, 12) centre (-41.5, 12) ccw
  line L1 (-41.5, 11) -> (-56.5, 11)
  line L2 (-56.5, 11) -> (-56.5, 5)
  line L3 (-56.5, 5) -> (-51.5, 5)
  line L4 (-51.5, 5) -> (-51.5, 9.5)
  line L5 (-51.5, 9.5) -> (-31, 9.5)
  line L6 (-31, 9.5) -> (-31, 19)
  line L7 (-31, 19) -> (-32.5, 19)
  arc A3 (-33.5, 18) -> (-32.5, 19) centre (-33.5, 19) ccw
  line L8 (-33.5, 18) -> (-39.5, 18)
  line L9 (-56.5, -5) -> (-56.5, 5)
  line L10 (-56.5, -5) -> (-51.5, -5)
  line L11 (-51.5, 5) -> (-51.5, -5)
  line L12 (-51.5, 5) -> (-56.5, 5)
extrude "Extrusion77" add sketch "Skizze69" against normal blind 10 contours L3 L9 L10 L11 L12 bodies 1
sketch "Skizze70" plane through (0, 0, -27.5) normal (0, 0, -1) x (-1, 0, 0)
  line L0 (-13, 2) -> (-13, 0)
  line L1 (-13, 0) -> (13, 0)
  line L2 (13, 0) -> (13, 2)
  line L3 (13, 2) -> (20.1, 2)
  line L4 (20.1, 2) -> (20.1, 9)
  line L5 (20.1, 9) -> (22, 9)
  line L6 (22, 9) -> (22, 0)
  line L7 (22, 0) -> (32.5, 0)
  line L8 (32.5, 0) -> (32.5, 19)
  line L9 (32.5, 19) -> (-32.5, 19)
  line L10 (-32.5, 19) -> (-32.5, 0)
  line L11 (-32.5, 0) -> (-22, 0)
  line L12 (-22, 0) -> (-22, 9)
  line L13 (-22, 9) -> (-20.1, 9)
  line L14 (-20.1, 9) -> (-20.1, 2)
  line L15 (-20.1, 2) -> (-13, 2)
  arc A0 (18.7617, 19) -> (-18.7617, 19) centre (0, 22) ccw
  circle A1 centre (0, 22) radius 19
  point P0 (-22, 44)
  point P1 (22, 44)
  constraint concentric A0 A1
extrude "Extrusion78" cut sketch "Skizze70" against normal blind 1.5 contours L9 A1 bodies 1
sketch "Skizze71" plane through (-57.5, 0, 0) normal (-1, 0, 0) x (0, 0, 1)
  line L0 (6.5, 19) -> (-6.5, 19)
  line L1 (-6.5, 19) -> (-6.5, 0)
  line L2 (-6.5, 0) -> (6.5, 0)
  line L3 (6.5, 0) -> (6.5, 19)
  circle A0 centre (0, 19) radius 4
  dimension "d349" = 8
  constraint midpoint L0 A0.centre
  measures "d349" diameter of A0
extrude "Extrusion79" cut sketch "Skizze71" against normal blind 6 contours L0 A0 | L0 A0 bodies 1 2
sketch "Skizze72" plane through (56.5, 0, 0) normal (1, 0, 0) x (0, 0, -1)
  line L0 (11, 24.5) -> (-11, 24.5)
  line L1 (-11, 24.5) -> (-11, 0)
  line L2 (-11, 0) -> (11, 0)
  line L3 (11, 0) -> (11, 24.5)
  circle A0 centre (0, 24.5) radius 4.5
  dimension "d352" = 9
  constraint midpoint L0 A0.centre
  measures "d352" diameter of A0
extrude "Extrusion80" cut sketch "Skizze72" against normal blind 5.5 contours L0 A0 | L0 A0 bodies 1 2
sketch "Skizze73" plane through (-32, 0, 32) normal (-0.707107, 0, 0.707107) x (0.707107, 0, 0.707107)
  line L0 (-19.7385, 19) -> (-14.8492, 19)
  line L1 (-14.8492, 19) -> (-14.8492, 33.5)
  line L2 (-14.8492, 33.5) -> (-15.5563, 33.5)
  line L3 (-15.5563, 33.5) -> (-15.5563, 47)
  line L4 (-15.5563, 47) -> (-36.0624, 47)
  line L5 (-36.0624, 47) -> (-36.0624, 19)
  line L6 (-36.0624, 19) -> (-23.2026, 19)
  arc A0 (-19.7385, 19) -> (-23.2026, 19) centre (-21.4706, 18) ccw
  line L7 (-23.2026, 19) -> (-19.7385, 19)
  constraint coincident L6.end A0.end
  constraint coincident L0.start A0.start
extrude "Extrusion81" add sketch "Skizze73" against normal blind 1.5 contours A0 L7 bodies 2
sketch "Skizze74" plane through (-32, 0, 32) normal (-0.707107, 0, 0.707107) x (0.707107, 0, 0.707107)
  line L0 (-36.0624, 19) -> (-14.8492, 19)
  line L1 (-14.8492, 19) -> (-14.8492, 33.5)
  line L2 (-14.8492, 33.5) -> (-15.5563, 33.5)
  line L3 (-15.5563, 33.5) -> (-15.5563, 47)
  line L4 (-15.5563, 47) -> (-36.0624, 47)
  line L5 (-36.0624, 47) -> (-36.0624, 19)
  circle A0 centre (-20.8492, 20.5) radius 1.5
  line L6 (-15.4706, 19) -> (-29.108, 19)
  line L7 (-19.3492, 20.5) -> (-19.3492, 19)
  line L8 (-22.3492, 20.5) -> (-22.3492, 19)
  dimension "d359" = 3
  dimension "d360" = 6
  constraint tangent L0 A0
  constraint coincident A0 L7.start
  constraint coincident L6 L7.end
  constraint perpendicular L0 L7
  constraint tangent A0 L7
  constraint coincident A0 L8.start
  constraint coincident L6 L8.end
  constraint perpendicular L0 L8
  constraint tangent A0 L8
  measures "d359" diameter of A0
  measures "d360" distance of L1 A0.centre
extrude "Extrusion82" cut sketch "Skizze74" against normal blind 1.5 contours L0 A0 L6 L8 | L0 A0 L6 L7 | A0 bodies 2
extrude "Extrusion83" add 4 faces at (-28.65, 10, -25.2151) (27.0473, 10, -25.2982) (28.65, 10, 25.2151) (-28.65, 10, 25.2151) along direction (0, 1, 0) blind 3 on bodies 1 bodies 1
extrude "Extrusion84" add 2 faces at (16, 44, -31.5333) (-16, 44, -35.5667) along direction (0, 1, 0) blind 3 on bodies 2 bodies 2
extrude "Extrusion85" cut 2 faces at (15.3333, 42, -34.5667) (-17.7, 42, -31.0333) along direction (0, 1, 0) blind 0.2 on bodies 2 bodies 2
sketch "Skizze75" plane through (0, 0, -39.6) normal (0, 0, -1) x (-1, 0, 0)
  line L0 (-22, 47) -> (-22, 35.2606)
  line L1 (-22, 35.2606) -> (-20, 35.2606)
  line L2 (-20, 35.2606) -> (-13, 42)
  line L3 (-13, 42) -> (-13, 47)
  line L4 (-13, 47) -> (-22, 47)
  line L5 (-13, 42.2) -> (-20, 35.2606)
  line L6 (13, 42.2) -> (20, 35)
  line L7 (13, 42) -> (20, 35)
  line L8 (20, 35) -> (22, 35)
  line L9 (22, 35) -> (22, 47)
  line L10 (22, 47) -> (13, 47)
  line L11 (13, 47) -> (13, 42)
  point P0 (-13, 42.2)
  point P1 (13, 42.2)
  point P2 (20, 35)
  constraint coincident P0 L5.start
  constraint coincident L1.end L2.start
  constraint coincident P1 L6.start
  constraint coincident P2 L6.end
extrude "Extrusion86" cut sketch "Skizze75" against normal blind 1.5 contours L2 L3 L5 | L6 L7 L11 bodies 2
extrude "Extrusion87" cut 4 faces at (39.6333, 33.5, 14.5) (39.6333, 33.5, -14.5) (-39.9603, 33.5, -24.3831) (-39.9603, 33.5, 24.3831) along direction (0, -1, 0) blind 3 on bodies 2 bodies 2
sketch "Skizze76" plane through (-32, 0, -32) normal (-0.707107, 0, -0.707107) x (-0.707107, 0, 0.707107)
  line L0 (15.5563, 47) -> (15.5563, 30.5)
  line L1 (15.5563, 30.5) -> (14.8492, 30.5)
  line L2 (14.8492, 30.5) -> (14.8492, 19)
  line L3 (14.8492, 19) -> (36.0624, 19)
  line L4 (36.0624, 19) -> (36.0624, 47)
  line L5 (36.0624, 47) -> (15.5563, 47)
  circle A0 centre (20.8492, 20.5) radius 1.5
  line L6 (22.3492, 20.5) -> (22.3492, 18.9)
  line L7 (19.3492, 20.5) -> (19.3492, 18.9)
  line L8 (14.8492, 19) -> (36.0624, 19)
  dimension "d373" = 3
  dimension "d374" = 6
  constraint tangent L3 A0
  constraint coincident A0 L6.start
  constraint tangent A0 L6
  constraint perpendicular L3 L6
  constraint coincident A0 L7.start
  constraint tangent A0 L7
  constraint perpendicular L3 L7
  measures "d373" diameter of A0
  measures "d374" distance of L2 A0.centre
extrude "Extrusion88" cut sketch "Skizze76" against normal blind 1.5 contours L3 A0 L6 L8 | L3 A0 L7 L8 | A0 bodies 2
sketch "Skizze77" plane through (0, 19, 0) normal (0, 1, 0) x (-1, 0, 0)
  line L0 (57.5, -4) -> (51.5218, -4)
  line L1 (51.5218, -4) -> (51.5218, -10.3569)
  line L2 (51.5218, -10.3569) -> (41.8787, -20)
  line L3 (41.8787, -20) -> (31, -20)
  line L4 (31, -20) -> (31, -26)
  line L5 (31, -26) -> (18.7617, -26)
  line L6 (18.7617, -26) -> (18.7617, -27.5)
  line L7 (18.7617, -27.5) -> (32.5, -27.5)
  line L8 (32.5, -27.5) -> (33.8276, -28.3587)
  arc A0 (33.8276, -28.3587) -> (39.5022, -26.9326) centre (36, -25) ccw
  line L9 (39.5022, -26.9326) -> (42.5, -21.5)
  line L10 (42.5, -21.5) -> (57.5, -6.5)
  line L11 (57.5, -6.5) -> (57.5, -4)
  circle A1 centre (36, -25) radius 1.9
  line L12 (41.8787, -20) -> (42.5, -21.5)
  line L13 (41.8787, 20) -> (42.5, 21.5)
  line L14 (31, -20) -> (31, 20)
  line L15 (51.5218, 4) -> (57.5, 4)
  line L16 (57.5, 4) -> (57.5, 6.5)
  line L17 (57.5, 6.5) -> (42.5, 21.5)
  line L18 (42.5, 21.5) -> (39.5022, 26.9326)
  arc A2 (39.5022, 26.9326) -> (33.8276, 28.3587) centre (36, 25) ccw
  line L19 (33.8276, 28.3587) -> (32.5, 27.5)
  line L20 (32.5, 27.5) -> (-32.5, 27.5)
  line L21 (-32.5, 27.5) -> (-32.5, 19)
  line L22 (-32.5, 19) -> (-31, 19)
  line L23 (-31, 19) -> (-31, 26)
  line L24 (-31, 26) -> (31, 26)
  line L25 (31, 26) -> (31, 20)
  line L26 (31, 20) -> (41.8787, 20)
  line L27 (41.8787, 20) -> (51.5218, 10.3569)
  line L28 (51.5218, 10.3569) -> (51.5218, 4)
  circle A3 centre (36, 25) radius 1.9
  line L29 (57.5, 4) -> (51.5218, 4)
  line L30 (51.5218, -4) -> (51.5218, 4)
  line L31 (51.5218, -4) -> (57.5, -4)
  line L32 (57.5, 4) -> (57.5, -4)
  line L33 (39.1754, -25) -> (37.5877, -22.25)
  line L34 (37.5877, -22.25) -> (34.4123, -22.25)
  line L35 (34.4123, -22.25) -> (32.8246, -25)
  line L36 (32.8246, -25) -> (34.4123, -27.75)
  line L37 (34.4123, -27.75) -> (37.5877, -27.75)
  line L38 (37.5877, -27.75) -> (39.1754, -25)
  line L39 (-32.8246, -14.5) -> (-34.4123, -11.75)
  line L40 (-34.4123, -11.75) -> (-37.5877, -11.75)
  line L41 (-37.5877, -11.75) -> (-39.1754, -14.5)
  line L42 (-39.1754, -14.5) -> (-37.5877, -17.25)
  line L43 (-37.5877, -17.25) -> (-34.4123, -17.25)
  line L44 (-34.4123, -17.25) -> (-32.8246, -14.5)
  line L45 (32.8246, 25) -> (34.4123, 22.25)
  line L46 (34.4123, 22.25) -> (37.5877, 22.25)
  line L47 (37.5877, 22.25) -> (39.1754, 25)
  line L48 (39.1754, 25) -> (37.5877, 27.75)
  line L49 (37.5877, 27.75) -> (34.4123, 27.75)
  line L50 (34.4123, 27.75) -> (32.8246, 25)
  line L51 (-32.8246, 14.5) -> (-34.4123, 17.25)
  line L52 (-34.4123, 17.25) -> (-37.5877, 17.25)
  line L53 (-37.5877, 17.25) -> (-39.1754, 14.5)
  line L54 (-39.1754, 14.5) -> (-37.5877, 11.75)
  line L55 (-37.5877, 11.75) -> (-34.4123, 11.75)
  line L56 (-34.4123, 11.75) -> (-32.8246, 14.5)
  arc A4 (-40.5, -17) -> (-39.5, -18) centre (-39.5, -17) ccw
  line L57 (-40.5, -17) -> (-40.5, -12)
  arc A5 (-40.5, -12) -> (-41.5, -11) centre (-41.5, -12) ccw
  line L58 (-41.5, -11) -> (-56.5, -11)
  line L59 (-56.5, -11) -> (-56.5, 11)
  line L60 (-56.5, 11) -> (-41.5, 11)
  arc A6 (-41.5, 11) -> (-40.5, 12) centre (-41.5, 12) ccw
  line L61 (-40.5, 12) -> (-40.5, 17)
  arc A7 (-39.5, 18) -> (-40.5, 17) centre (-39.5, 17) ccw
  line L62 (-39.5, 18) -> (-33.5, 18)
  arc A8 (-33.5, 18) -> (-32.5, 19) centre (-33.5, 19) ccw
  line L63 (-32.5, 19) -> (-32.5, 27.5)
  line L64 (-32.5, 27.5) -> (32.5, 27.5)
  line L65 (32.5, 27.5) -> (33.8276, 28.3587)
  arc A9 (39.5022, 26.9326) -> (33.8276, 28.3587) centre (36, 25) ccw
  line L66 (39.5022, 26.9326) -> (42.5, 21.5)
  line L67 (42.5, 21.5) -> (57.5, 6.5)
  line L68 (57.5, 6.5) -> (57.5, -6.5)
  line L69 (57.5, -6.5) -> (42.5, -21.5)
  line L70 (42.5, -21.5) -> (39.5022, -26.9326)
  arc A10 (33.8276, -28.3587) -> (39.5022, -26.9326) centre (36, -25) ccw
  line L71 (33.8276, -28.3587) -> (32.5, -27.5)
  line L72 (32.5, -27.5) -> (22, -27.5)
  line L73 (22, -27.5) -> (22, -39.6)
  line L74 (22, -39.6) -> (13, -39.6)
  line L75 (13, -39.6) -> (13, -27.5)
  line L76 (13, -27.5) -> (-13, -27.5)
  line L77 (-13, -27.5) -> (-13, -39.6)
  line L78 (-13, -39.6) -> (-22, -39.6)
  line L79 (-22, -39.6) -> (-22, -27.5)
  line L80 (-22, -27.5) -> (-32.5, -27.5)
  line L81 (-32.5, -27.5) -> (-32.5, -19)
  arc A11 (-32.5, -19) -> (-33.5, -18) centre (-33.5, -19) ccw
  line L82 (-33.5, -18) -> (-39.5, -18)
  point P0 (41.8787, 20)
  point P1 (42.5, 21.5)
  point P2 (31, 20)
  constraint coincident L2.end L3.start
  constraint coincident L9.end L10.start
  constraint coincident P0 L13.start
  constraint coincident P1 L13.end
  constraint coincident L3.end L4.start
  constraint coincident P2 L14.end
extrude "Extrusion89" cut sketch "Skizze77" against normal blind 19 contours L0 L1 L2 L10 L11 L12 L31 L68 L69 | L0 L15 L29 L30 L31 L32 L68 | L1 L2 L3 L14 L26 L27 L28 L30 | L13 L15 L16 L17 L27 L28 L29 L67 L68 bodies 1
sketch "Skizze78" plane through (0, 3, 0) normal (0, 1, 0) x (-1, 0, 0)
  line L0 (31, -20) -> (31, 20)
  line L1 (31, 20) -> (31, 22)
  arc A0 (23, 22) -> (31, 22) centre (27, 22) ccw
  line L2 (23, 22) -> (23, 26)
  line L3 (23, 26) -> (-23, 26)
  line L4 (-23, 26) -> (-23, 22)
  arc A1 (-31, 22) -> (-23, 22) centre (-27, 22) ccw
  line L5 (-31, 22) -> (-31, 9.5)
  line L6 (-31, 9.5) -> (-51.5, 9.5)
  line L7 (-51.5, 9.5) -> (-51.5, -9.5)
  line L8 (-51.5, -9.5) -> (-31, -9.5)
  line L9 (-31, -9.5) -> (-31, -22)
  arc A2 (-23, -22) -> (-31, -22) centre (-27, -22) ccw
  line L10 (-23, -22) -> (-23, -26)
  line L11 (-23, -26) -> (0, -26)
  line L12 (0, -26) -> (23, -26)
  line L13 (23, -26) -> (23, -22)
  arc A3 (31, -22) -> (23, -22) centre (27, -22) ccw
  line L14 (31, -22) -> (31, -20)
  arc A4 (31, 20) -> (31, -20) centre (45.151, 0) ccw
  line L15 (24, 22) -> (23, 22)
  arc A5 (23, 22) -> (31, 22) centre (27, 22) ccw
  line L16 (31, 22) -> (30, 22)
  arc A6 (24, 22) -> (30, 22) centre (27, 22) ccw
  line L17 (30, -22) -> (31, -22)
  arc A7 (31, -22) -> (23, -22) centre (27, -22) ccw
  line L18 (23, -22) -> (24, -22)
  arc A8 (30, -22) -> (24, -22) centre (27, -22) ccw
  line L19 (31, -20) -> (31, 20)
  dimension "d379" = 24.5
  constraint coincident L0.end L1.start
  constraint coincident L0.start L14.end
  measures "d379" radius of A4
extrude "Extrusion90" cut sketch "Skizze78" against normal blind 3 contours L0 A4 L19 bodies 1
sketch "Skizze79" plane through (0, 19, 0) normal (0, 1, 0) x (-1, 0, 0)
  circle A0 centre (36, 25) radius 1.9
  line L0 (41.8787, 20) -> (42.5, 21.5)
  line L1 (42.5, 21.5) -> (39.5022, 26.9326)
  arc A1 (39.5022, 26.9326) -> (33.8276, 28.3587) centre (36, 25) ccw
  line L2 (33.8276, 28.3587) -> (32.5, 27.5)
  line L3 (32.5, 27.5) -> (-32.5, 27.5)
  line L4 (-32.5, 27.5) -> (-32.5, 19)
  line L5 (-32.5, 19) -> (-31, 19)
  line L6 (-31, 19) -> (-31, 26)
  line L7 (-31, 26) -> (31, 26)
  line L8 (31, 26) -> (31, 20)
  line L9 (31, 20) -> (41.8787, 20)
  line L10 (42.5, -21.5) -> (41.8787, -20)
  line L11 (41.8787, -20) -> (31, -20)
  line L12 (31, -20) -> (31, -26)
  line L13 (31, -26) -> (18.7617, -26)
  line L14 (18.7617, -26) -> (18.7617, -27.5)
  line L15 (18.7617, -27.5) -> (32.5, -27.5)
  line L16 (32.5, -27.5) -> (33.8276, -28.3587)
  arc A2 (33.8276, -28.3587) -> (39.5022, -26.9326) centre (36, -25) ccw
  line L17 (39.5022, -26.9326) -> (42.5, -21.5)
  circle A3 centre (36, -25) radius 1.9
  circle A4 centre (36, 25) radius 4
  circle A5 centre (36, -25) radius 4
  arc A6 (36.0513, 21.0003) -> (31, 20) centre (36.233, 6.8289) ccw
  line L18 (-1.75, 0) -> (-22.5, 0)
  arc A7 (31, -20) -> (36.0513, -21.0003) centre (36.233, -6.8289) ccw
  constraint concentric A0 A4
  constraint concentric A2 A5
  constraint tangent A1 A4
  constraint tangent A2 A5
  constraint coincident A4 A6.start
  constraint coincident L8.end L9.start
  constraint tangent A4 A6
  constraint symmetric L8.end L18 L11.end
  constraint symmetric A6.start L18 A7.end
  constraint symmetric A6 L18 A7
extrude "Extrusion91" cut sketch "Skizze79" against normal blind 19 contours L0 L1 L9 A4 A6 | L10 L11 L17 A5 A7 bodies 1
extrude "Extrusion92" cut 2 faces at (-33.8417, 3, -23.8085) (-33.8417, 3, 26.1915) along direction (0, 1, 0) blind 10 on bodies 1 bodies 1
sketch "Skizze80" plane through (0, 0, 0) normal (0, -1, 0) x (1, 0, 0)
  arc A0 (-36.0513, -21.0003) -> (-33.8276, -28.3587) centre (-36, -25) ccw
  line L0 (-33.8276, -28.3587) -> (-32.5, -27.5)
  line L1 (-32.5, -27.5) -> (-22, -27.5)
  line L2 (-22, -27.5) -> (-22, -39.6)
  line L3 (-22, -39.6) -> (-13, -39.6)
  line L4 (-13, -39.6) -> (-13, -27.5)
  line L5 (-13, -27.5) -> (13, -27.5)
  line L6 (13, -27.5) -> (13, -39.6)
  line L7 (13, -39.6) -> (22, -39.6)
  line L8 (22, -39.6) -> (22, -27.5)
  line L9 (22, -27.5) -> (32.5, -27.5)
  line L10 (32.5, -27.5) -> (32.5, -19)
  arc A1 (33.5, -18) -> (32.5, -19) centre (33.5, -19) ccw
  line L11 (33.5, -18) -> (39.5, -18)
  arc A2 (39.5, -18) -> (40.5, -17) centre (39.5, -17) ccw
  line L12 (40.5, -17) -> (40.5, -12)
  arc A3 (41.5, -11) -> (40.5, -12) centre (41.5, -12) ccw
  line L13 (41.5, -11) -> (56.5, -11)
  line L14 (56.5, -11) -> (56.5, 11)
  line L15 (56.5, 11) -> (41.5, 11)
  arc A4 (40.5, 12) -> (41.5, 11) centre (41.5, 12) ccw
  line L16 (40.5, 12) -> (40.5, 17)
  arc A5 (40.5, 17) -> (39.5, 18) centre (39.5, 17) ccw
  line L17 (39.5, 18) -> (33.5, 18)
  arc A6 (32.5, 19) -> (33.5, 18) centre (33.5, 19) ccw
  line L18 (32.5, 19) -> (32.5, 27.5)
  line L19 (32.5, 27.5) -> (-32.5, 27.5)
  line L20 (-32.5, 27.5) -> (-33.8276, 28.3587)
  arc A7 (-33.8276, 28.3587) -> (-36.0513, 21.0003) centre (-36, 25) ccw
  arc A8 (-31, 20) -> (-36.0513, 21.0003) centre (-36.233, 6.8289) ccw
  arc A9 (-31, -20) -> (-31, 20) centre (-45.151, 0) ccw
  arc A10 (-36.0513, -21.0003) -> (-31, -20) centre (-36.233, -6.8289) ccw
  line L21 (-39.1754, -25) -> (-37.5877, -22.25)
  line L22 (-37.5877, -22.25) -> (-34.4123, -22.25)
  line L23 (-34.4123, -22.25) -> (-32.8246, -25)
  line L24 (-32.8246, -25) -> (-34.4123, -27.75)
  line L25 (-34.4123, -27.75) -> (-37.5877, -27.75)
  line L26 (-37.5877, -27.75) -> (-39.1754, -25)
  line L27 (32.8246, -14.5) -> (34.4123, -11.75)
  line L28 (34.4123, -11.75) -> (37.5877, -11.75)
  line L29 (37.5877, -11.75) -> (39.1754, -14.5)
  line L30 (39.1754, -14.5) -> (37.5877, -17.25)
  line L31 (37.5877, -17.25) -> (34.4123, -17.25)
  line L32 (34.4123, -17.25) -> (32.8246, -14.5)
  line L33 (-32.8246, 25) -> (-34.4123, 22.25)
  line L34 (-34.4123, 22.25) -> (-37.5877, 22.25)
  line L35 (-37.5877, 22.25) -> (-39.1754, 25)
  line L36 (-39.1754, 25) -> (-37.5877, 27.75)
  line L37 (-37.5877, 27.75) -> (-34.4123, 27.75)
  line L38 (-34.4123, 27.75) -> (-32.8246, 25)
  line L39 (32.8246, 14.5) -> (34.4123, 17.25)
  line L40 (34.4123, 17.25) -> (37.5877, 17.25)
  line L41 (37.5877, 17.25) -> (39.1754, 14.5)
  line L42 (39.1754, 14.5) -> (37.5877, 11.75)
  line L43 (37.5877, 11.75) -> (34.4123, 11.75)
  line L44 (34.4123, 11.75) -> (32.8246, 14.5)
  circle A11 centre (-36, 25) radius 4
  circle A12 centre (-36, -25) radius 4
  line L45 (-32.5, -27.5) -> (-32.6769, -27.2265)
  line L46 (-34.4939, -20.8944) -> (-34.4939, -21.2944)
  line L47 (0, 1.75) -> (0, 22.5)
  line L48 (-32.5, 27.5) -> (-32.6769, 27.2265)
  line L49 (-34.4939, 21.2944) -> (-34.4939, 20.8944)
  dimension "d386" = 0.4
  dimension "d387" = 0.4
  constraint concentric A7 A11
  constraint concentric A0 A12
  constraint tangent A0 A12
  constraint tangent A7 A11
  constraint coincident L0.end L1.start
  constraint coincident A12 L45.end
  constraint perpendicular L0 L45
  constraint coincident A10 L46.start
  constraint coincident A12 L46.end
  constraint parallel L46 L47
  constraint coincident L19.end L20.start
  constraint coincident A11 L48.end
  constraint perpendicular L20 L48
  constraint coincident A11 L49.start
  constraint coincident A8 L49.end
  constraint parallel L47 L49
  measures "d386" vertical distance of L46.start L46.end
  measures "d387" vertical distance of L49.start L49.end
extrude "Extrusion93" cut sketch "Skizze80" against normal blind 10 contours A0 A12 | A10 A12 L46 | L0 A12 L45 | A8 A11 L49 | A7 A11 | L20 A11 L48 bodies 1